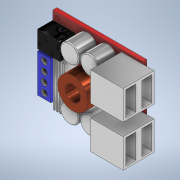
# Autodesk Inventor part: Step_Down_USB
Saved by Autodesk Inventor 2021 (Build 250183000, 183)
## iProperties
Created: 2021-07-29
Part Number: Step_Down_USB
Material: Generisch
Document SubType Name: Modeling
Designer: User
Density: 1 g/cm^3
Appearance: Vorgabe
Author: User
Autodesk Inventor part; units mm, degrees
ref_plane "YZ Plane" through (0, 0, 0) normal (1, 0, 0) x (0, 1, 0)
ref_plane "XZ Plane" through (0, 0, 0) normal (0, 1, 0) x (-1, 0, 0)
ref_plane "XY Plane" through (0, 0, 0) normal (0, 0, 1) x (1, 0, 0)
sketch "Skizze1" plane through (0, 0, 0) normal (0, 0, 1) x (1, 0, 0)
  line L0 (-23.5, 19.5) -> (23.5, 19.5)
  line L1 (23.5, 19.5) -> (23.5, -19.5)
  line L2 (23.5, -19.5) -> (-23.5, -19.5)
  line L3 (-23.5, -19.5) -> (-23.5, 19.5)
  line L4 (-23.5, -19.5) -> (23.5, 19.5) construction
  circle A0 centre (-21.0614, 17.0614) radius 1
  circle A1 centre (16, 0) radius 1.5
  line L5 (-23.5, 0) -> (23.5, 0) construction
  circle A2 centre (-21.0614, -17.0614) radius 1
  line L6 (-21.0614, -17.0614) -> (-21.0614, 17.0614) construction
  line L7 (-23.5, 19.5) -> (-21.0614, 17.0614) construction
  line L8 (12.5, -18.5) -> (29.5, -18.5)
  line L9 (29.5, -18.5) -> (29.5, -3.3)
  line L10 (29.5, -3.3) -> (12.5, -3.3)
  line L11 (12.5, -3.3) -> (12.5, -18.5)
  line L12 (12.5, 3.3) -> (29.5, 3.3)
  line L13 (29.5, 3.3) -> (29.5, 18.5)
  line L14 (29.5, 18.5) -> (12.5, 18.5)
  line L15 (12.5, 18.5) -> (12.5, 3.3)
  circle A3 centre (-5.25, -13.5) radius 5
  circle A4 centre (5.25, -13.5) radius 5
  circle A5 centre (-5.25, 13.5) radius 5
  circle A6 centre (5.25, 13.5) radius 5
  circle A7 centre (0, 0) radius 8
  circle A8 centre (0, 0) radius 4
  line L16 (-23.4, 5.9386) -> (-11.75, 5.9386)
  line L17 (-11.75, 5.9386) -> (-11.75, 14.9386)
  line L18 (-11.75, 14.9386) -> (-23.4, 14.9386)
  line L19 (-23.4, 14.9386) -> (-23.4, 5.9386)
  line L20 (-23.4, -15.0614) -> (-16.4, -15.0614)
  line L21 (-16.4, -15.0614) -> (-16.4, 4.9386)
  line L22 (-16.4, 4.9386) -> (-23.4, 4.9386)
  line L23 (-23.4, 4.9386) -> (-23.4, -15.0614)
  line L24 (0, 19.5) -> (0, -19.5) construction
  line L25 (-16.3, -18.5) -> (-10.5, -18.5)
  line L26 (-10.5, -18.5) -> (-10.5, 4.9386)
  line L27 (-10.5, 4.9386) -> (-16.3, 4.9386)
  line L28 (-16.3, 4.9386) -> (-16.3, -18.5)
  dimension "d0" = 39
  dimension "d1" = 47
  dimension "d2" = 3
  dimension "d3" = 2
  dimension "d4" = 38.3
  dimension "d5" = 6
  dimension "d6" = 45
  dimension "d7" = 10
  dimension "d8" = 0.5
  dimension "d9" = 1
  dimension "d10" = 16
  dimension "d11" = 15.2
  dimension "d13" = 6
  dimension "d14" = 17
  dimension "d15" = 15.2
  dimension "d16" = 1
  dimension "d17" = 8
  dimension "d18" = 20
  dimension "d19" = 7
  dimension "d20" = 0.1
  dimension "d21" = 5.8
  dimension "d22" = 0.1
  dimension "d23" = 1
  dimension "d24" = 1
  dimension "d25" = 0.1
  dimension "d26" = 9
  dimension "d27" = 1
  dimension "d28" = 1.5
  constraints: 58 end point, 12 parallel, 9 centre point, 7 perpendicular, 6 horizontal, 5 midpoint, 4 equal radius, 4 symmetric about line, 3 coincident, 2 collinear, 2 point on line, 1 other
  measures "d0" distance of L2.end L0.start
  measures "d1" distance of L0.start L0.end
  measures "d2" diameter of A1
  measures "d3" diameter of A0
  measures "d5" distance edge to line of A1 L1
  measures "d6" angle of L7 L0
  measures "d7" diameter of A5
  measures "d9" distance edge to line of A4 L2
  measures "d10" diameter of A7
  measures "d11" distance between parallel lines of L10 L8
  measures "d13" distance between parallel lines of L9 L1
  measures "d14" distance of L8.start L8.end
  measures "d15" distance of L12.end L13.end
  measures "d16" distance between parallel lines of L8 L2
  measures "d17" diameter of A8
  measures "d18" distance of L22.end L20.start
  measures "d19" distance of L20.start L20.end
  measures "d20" distance between parallel lines of L21 L28
  measures "d21" distance between parallel lines of L28 L26
  measures "d22" distance between parallel lines of L3 L23
  measures "d23" distance between parallel lines of L25 L2
  measures "d24" distance edge to line of A2 L20
  measures "d25" distance between parallel lines of L3 L19
  measures "d26" distance between parallel lines of L18 L16
  measures "d27" distance between parallel lines of L16 L22
  measures "d28" distance edge to line of A5 L17
extrude "Extrusion1" add sketch "Skizze1" against normal blind 2.2 contours L0 L1 L14 L15 L12 L10 L11 L8 L2 L3 | L1 L12 L15 L14 | L8 L11 L10 L1 | A3 | A4 | A5 | A6 | A7 | A8 | L19 L18 L17 L16 | L23 L22 L21 L20 | L28 L27 L26 L25
extrude "Extrusion2" add sketch "Skizze1" along normal blind 16.2 contours L14 L13 L12 L1 | L1 L12 L15 L14 | L8 L11 L10 L1 | L1 L10 L9 L8
sketch "Skizze2" plane through (29.5, -18.5, 0) normal (1, 0, 0) x (0, 0, -1)
  line L0 (-14.8, 1.2) -> (-9.5, 1.2)
  line L1 (-9.5, 1.2) -> (-9.5, 14)
  line L2 (-9.5, 14) -> (-14.8, 14)
  line L3 (-14.8, 14) -> (-14.8, 1.2)
  line L4 (-6.4, 1.2) -> (-1.1, 1.2)
  line L5 (-1.1, 1.2) -> (-1.1, 14)
  line L6 (-1.1, 14) -> (-6.4, 14)
  line L7 (-6.4, 14) -> (-6.4, 1.2)
  line L8 (0, 0) -> (0, 15.2) projected
  line L9 (-16.2, 15.2) -> (-16.2, 0) projected
  line L10 (-16.2, 7.6) -> (0, 7.6) construction
  line L11 (0, 38) -> (0, -1) projected
  point P0 (0, 18.5)
  dimension "d33" = 1.1
  dimension "d34" = 5.3
  dimension "d35" = 5.3
  dimension "d36" = 3.1
  dimension "d37" = 12.8
  constraints: 18 end point, 4 parallel, 3 perpendicular, 3 point on line, 2 horizontal, 1 midpoint, 1 other
  measures "d33" distance between parallel lines of L5 L8
  measures "d34" distance of L4.start L4.end
  measures "d35" distance of L0.start L0.end
  measures "d36" distance between parallel lines of L1 L7
  measures "d37" distance between parallel lines of L0 L2
extrude "Extrusion3" cut sketch "Skizze2" against normal blind 10
extrude "Extrusion4" add sketch "Skizze1" along normal blind 9.5 contours A3 | A4
mirror "Spiegeln1" about plane through (0, 0, 0) normal (0, 1, 0) of "Extrusion4", "Extrusion3"
extrude "Extrusion5" add sketch "Skizze1" along normal blind 13 contours A7
extrude "Extrusion6" add sketch "Skizze1" along normal blind 8 contours L23 L22 L21 L20
extrude "Extrusion11" add sketch "Skizze1" along normal blind 8 contours L19 L18 L17 L16
extrude "Extrusion7" add sketch "Skizze1" along normal blind 7 contours L28 L27 L26 L25
sketch "Skizze3" plane through (-16.3, -18.5, 0) normal (0, -1, 0) x (1, 0, 0)
  line L0 (0, 7) -> (5.8, 7) projected
  line L1 (0.8004, 7) -> (0.8004, 0.8568)
  line L2 (0.8004, 0.8568) -> (1.6289, 0.8568)
  line L3 (1.6289, 0.8568) -> (1.6289, 7)
  line L4 (2.4575, 7) -> (2.4575, 0.8568)
  line L5 (2.4575, 0.8568) -> (3.2861, 0.8568)
  line L6 (3.2861, 0.8568) -> (3.2861, 7)
  line L7 (4.1146, 7) -> (4.1146, 0.8568)
  line L8 (4.1146, 0.8568) -> (4.9432, 0.8568)
  line L9 (4.9432, 0.8568) -> (4.9432, 7)
  line L10 (0, 0) -> (0, 7) projected
  line L11 (5.8, 0) -> (5.8, 7) projected
  point P0 (16.3, 0)
  dimension "d48" = 5.8
  dimension "d49" = 0.8286
  dimension "d50" = 0.8286
  dimension "d51" = 0.8286
  constraints: 18 end point, 10 point on line, 5 perpendicular, 2 collinear, 1 parallel, 1 vertical
  measures "d48" distance between parallel lines of L10 L11
  measures "d49" distance between parallel lines of L3 L1
  measures "d50" distance between parallel lines of L3 L4
  measures "d51" distance between parallel lines of L7 L6
extrude "Extrusion8" cut sketch "Skizze3" against normal up to surface (23.4386 mm away)
fillet "Rundung1" radius 0.5 4 edges at (-10.25, -13.5, 9.5) (0.25, -13.5, 9.5) (-10.25, 13.5, 9.5) (0.25, 13.5, 9.5)
sketch "Skizze4" plane through (0, 0, 8) normal (0, 0, 1) x (1, 0, 0)
  circle A0 centre (-19.9, 2.1386) radius 1.6
  circle A1 centre (-19.9, -2.6614) radius 1.6
  circle A2 centre (-19.9, -7.4614) radius 1.6
  circle A3 centre (-19.9, -12.2614) radius 1.6
  line L0 (-16.4, 4.9386) -> (-23.4, 4.9386) projected
  line L1 (-19.9, 4.9386) -> (-19.9, -15.0614) construction
  line L2 (-16.4, -15.0614) -> (-23.4, -15.0614) projected
  line L3 (-23.4, -15.0614) -> (-23.4, 4.9386) projected
  line L4 (-23.4, -5.0614) -> (-16.4, -5.0614) construction
  point P0 (0, 0)
  dimension "d55" = 3.2
  dimension "d56" = 4.8
  dimension "d57" = 4.8
  dimension "d58" = 4.8
  constraints: 4 centre point, 4 end point, 4 point on line, 3 equal radius, 3 midpoint, 1 horizontal, 1 other
  measures "d55" diameter of A0
  measures "d56" distance of A1.centre A0.centre
  measures "d57" distance of A1.centre A2.centre
  measures "d58" distance of A2.centre A3.centre
extrude "Extrusion9" cut sketch "Skizze4" against normal up to surface (8 mm away)
sketch "Skizze5" plane through (-23.4, -15.0614, 0) normal (-1, 0, 0) x (0, 0, 1)
  line L0 (0.5, 19.15) -> (5, 19.15)
  line L1 (5, 19.15) -> (5, 15.25)
  line L2 (5, 15.25) -> (0.5, 15.25)
  line L3 (0.5, 15.25) -> (0.5, 19.15)
  line L4 (0.5, 14.35) -> (5, 14.35)
  line L5 (5, 14.35) -> (5, 10.45)
  line L6 (5, 10.45) -> (0.5, 10.45)
  line L7 (0.5, 10.45) -> (0.5, 14.35)
  line L8 (0.5, 5.65) -> (5, 5.65)
  line L9 (5, 5.65) -> (5, 9.55)
  line L10 (5, 9.55) -> (0.5, 9.55)
  line L11 (0.5, 9.55) -> (0.5, 5.65)
  line L12 (0.5, 4.75) -> (5, 4.75)
  line L13 (5, 4.75) -> (5, 0.85)
  line L14 (5, 0.85) -> (0.5, 0.85)
  line L15 (0.5, 0.85) -> (0.5, 4.75)
  line L16 (8, 17.2) -> (5, 17.2) construction
  line L17 (0.5, 17.2) -> (5, 17.2) construction
  line L18 (0.5, 12.4) -> (5, 12.4) construction
  line L19 (8, 12.4) -> (5, 12.4) construction
  line L20 (8, 7.6) -> (5, 7.6) construction
  line L21 (0.5, 7.6) -> (5, 7.6) construction
  line L22 (8, 20) -> (8, 0) construction
  line L23 (0.5, 2.8) -> (5, 2.8) construction
  line L24 (5, 2.8) -> (8, 2.8) construction
  line L25 (0, 34.5614) -> (0, -4.4386) construction
  circle A0 centre (4, 25.5) radius 2.5
  line L26 (4, 30) -> (4, 21) construction
  line L27 (8, 25.5) -> (0, 25.5) construction
  line L28 (0, 30) -> (8, 30) projected
  line L29 (8, 30) -> (8, 21) projected
  line L30 (0, 21) -> (8, 21) projected
  line L31 (0, 21) -> (0, 30) projected
  point P0 (0, 15.0614)
  point P1 (4, 25.5)
  dimension "d61" = 0.5
  dimension "d62" = 4.5
  dimension "d63" = 3.9
  dimension "d66" = 5
  constraints: 52 end point, 13 midpoint, 8 parallel, 7 perpendicular, 6 point on line, 4 collinear, 4 equal length, 4 horizontal, 1 centre point, 1 coincident
  measures "d61" distance between parallel lines of L25 L3
  measures "d62" distance between parallel lines of L1 L3
  measures "d63" distance of L0.end L1.end
  measures "d66" diameter of A0
extrude "Extrusion10" cut sketch "Skizze5" against normal blind 7 contours L0 L1 L2 L3 | L4 L5 L6 L7 | L11 L10 L9 L8 | L12 L13 L14 L15 | A0
equation "\"d15\" = d11"
